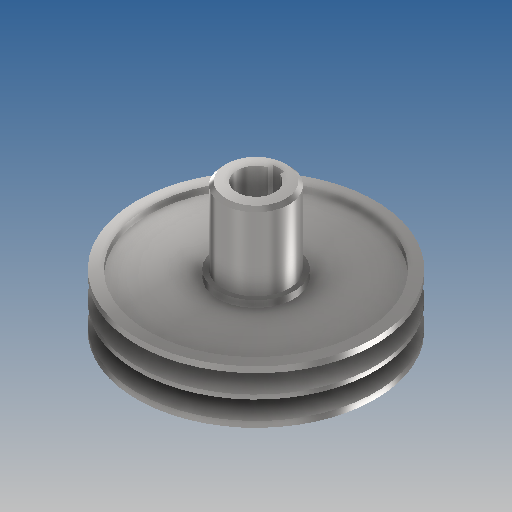
# Autodesk Inventor part: PWTR-0094
Saved by Autodesk Inventor 2021.1 (Build 251245000, 245)
## iProperties
Created: 2020-08-28
Part Number: PWTR-0094
Material: Stainless Steel
Document SubType Name: Modeling
Designer: alid
Density: 8 g/cm^3
Appearance: Semi-Polished
Description: Drive Unit Lower Pulley
Author: alid
Revision Number: A
Autodesk Inventor part; units mm, degrees
ref_plane "YZ Plane" through (0, 0, 0) normal (1, 0, 0) x (0, 1, 0)
ref_plane "XZ Plane" through (0, 0, 0) normal (0, 1, 0) x (-1, 0, 0)
sketch "Sketch1" plane through (0, 0, 0) normal (0, 0, 1) x (1, 0, 0)
  circle A0 centre (0, 0) radius 10
  circle A1 centre (0, 0) radius 17.5
  line L0 (-3, 9.5394) -> (-3, 12)
  line L1 (-3, 12) -> (3, 12)
  line L2 (3, 12) -> (3, 9.5394)
  line L3 (-8.124, -15.5) -> (8.124, -15.5)
  dimension "d0" = 20
  dimension "d1" = 35
  dimension "d2" = 12
  dimension "d3" = 6
  dimension "d4" = 15.5
  constraints: 8 end point, 4 point on circle, 2 centre point, 2 coincident, 2 perpendicular, 1 horizontal, 1 parallel, 1 vertical
  measures "d0" diameter of A0
  measures "d1" diameter of A1
  measures "d2" distance from line of point (0, 0) L1
  measures "d3" distance of L0.end L1.end
  measures "d4" distance from line of point (0, 0) L3
extrude "Extrusion1" add sketch "Sketch1" along normal mid plane 40 contours A0 | A0 L0 L1 L2 | A1 L3 | L3 A1
extrude "Extrusion2" [suppressed]
chamfer "Chamfer1" [suppressed]
sketch "Sketch2" plane through (0, 0, 0) normal (0, 1, 0) x (-1, 0, 0)
  line L0 (0, 10) -> (0, -10)
  point P0 (0, 0)
  point P1 (0, 0)
  dimension "d12" = 20
  constraints: 2 end point, 1 coincident, 1 midpoint, 1 vertical
  measures "d12" distance of L0.start L0.end
hole "Hole1" [suppressed]
sketch "Sketch3" plane through (0, 0, -20) normal (0, 0, -1) x (-1, 0, 0)
  circle A0 centre (0, 0) radius 17.5 projected
  circle A1 centre (0, 0) radius 62.5
  circle A2 centre (0, 0) radius 20
  circle A3 centre (0, 0) radius 56.5
  dimension "d32" = 125
  dimension "d45" = 6
  dimension "d46" = 40
  constraints: 3 centre point, 3 coincident
  measures "d32" diameter of A1
  measures "d45" radial gap between concentric circles of A1 A3
  measures "d46" diameter of A2
extrude "Extrusion3" add sketch "Sketch3" along normal blind 28 contours A0 | A1 | A2 | A3
ref_plane "Work Plane1" through (0, 0, -34) normal (0, 0, 1) x (1, 0, 0)
extrude "Extrusion4" cut sketch "Sketch3" along normal blind 3.5 contours A3
mirror "Mirror1" about plane through (0, 0, -34) normal (0, 0, 1) of "Extrusion4"
sketch "Sketch4" plane through (0, 0, -48) normal (0, 0, -1) x (-1, 0, 0)
  point P0 (0, 0)
  point P1 (0, 0)
  point P2 (0, 0)
  constraints: 1 coincident
hole "Hole2" at (0, 0, -48) direction (0, 0, 1) diameter 6.6 end through all counterbore diameter 11 counterbore depth 20 clearance for "Socket Head Cap Screw ISO 4762" size "M6" standard "ISO"
chamfer "Chamfer2" distance 1.75 angle 45 1 edges at (-17.5, 0, 20)
sketch "Sketch5" plane through (0, 0, 0) normal (1, 0, 0) x (0, 1, 0)
  line L0 (62.5, -23.137) -> (51.5, -26.5)
  line L1 (51.5, -26.5) -> (51.5, -29.5)
  line L2 (51.5, -29.5) -> (62.5, -32.863)
  line L3 (51.5, -28) -> (62.5, -28) construction
  line L4 (62.5, -23.137) -> (62.5, -32.863)
  line L5 (62.5, -20) -> (62.5, -48) projected
  line L6 (0, -57.6) -> (0, 9.6) projected
  point P0 (0, 0)
  dimension "d34" = 34
  dimension "d35" = 11
  dimension "d39" = 3
  dimension "d40" = 8
  constraints: 10 end point, 2 midpoint, 1 perpendicular, 1 point on line, 1 other
  measures "d34" angle of L0 L2
  measures "d35" distance between parallel lines of L1 L4
  measures "d39" distance of L0.end L1.end
  measures "d40" distance from line of L5.start L3
revolve "Revolution1" cut sketch "Sketch5" angle 360 about axis through (0, 0, -10) along (0, 0, 1)
pattern_linear "Rectangular Pattern1" count 2 spacing 12 along (0, 0, -1) of "Revolution1"
extrude "Extrusion5" cut sketch "Sketch1" along normal through all contours A0 | A0 L0 L1 L2
chamfer "Chamfer3" distance 1.75 angle 45 1 edges at (0, -5.5, -48)
equation "\"d34\" = d37"
equation "\"d35\" = d38"
equation "\"d36\" = 8.5"
equation "\"d37\" = 34deg"
equation "\"d38\" = 11"
body "Solid1"
